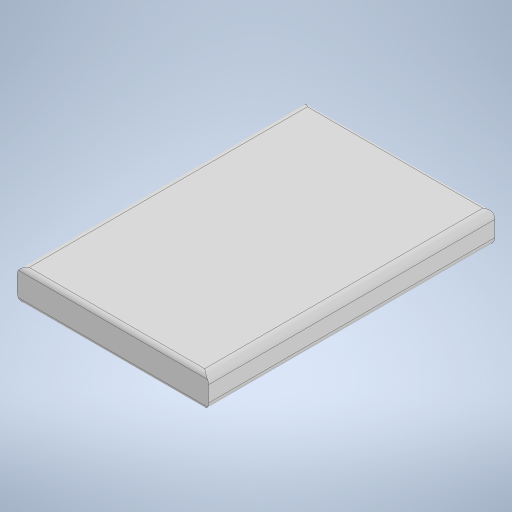
# Autodesk Inventor part: Battery_402535
Saved by Autodesk Inventor 2023 (Build 270158000, 158)
## iProperties
Created: 2023-03-12
Part Number: Battery_402535
Material: Generic
Document SubType Name: Modeling
Designer: nigel
Density: 1 g/cm^3
Appearance: Default
Author: nigel
Autodesk Inventor part; units mm, degrees
ref_plane "YZ Plane" through (0, 0, 0) normal (1, 0, 0) x (0, 1, 0)
sketch "Sketch1" plane through (0, 0, 0) normal (0, 1, 0) x (-1, 0, 0)
  line L0 (0, 0) -> (-24.2, 0)
  line L1 (-24.2, 0) -> (-24.2, -36.2)
  line L2 (-24.2, -36.2) -> (0, -36.2)
  line L3 (0, -36.2) -> (0, 0)
  dimension "d0" = 24.2
  dimension "d1" = 36.2
  constraints: 8 end point, 2 parallel, 1 horizontal, 1 perpendicular
  measures "d0" distance of L1.end L2.end
  measures "d1" distance of L2.end L0.start
extrude "Extrusion1" add sketch "Sketch1" along normal blind 4
fillet "Fillet1" radius 1 4 edges at (0, 4, -18.1) (0, 0, -18.1) (24.2, 4, -18.1) (24.2, 0, -18.1)
fillet "Fillet1" radius 0.5 4 edges at (12.1, 4, -36.2) (12.1, 0, -36.2) (12.1, 4, 0) (12.1, 0, 0)
ref_plane "Work Plane1" through (12.1, 1, -36.2) normal (1, 0, 0) x (0, 0, -1)
ref_plane "Work Plane2" through (0.134, 3.5, -18.1) normal (0, 0, 1) x (1, 0, 0)
body "Solid1"
